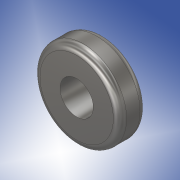
# Autodesk Inventor part: 10x26x8 Bearing
Saved by Autodesk Inventor 2017 SP1 (Build 210196100, 196)
## iProperties
Created: 2017-07-03
Part Number: 10x26x8 Bearing
Material: Steel, Carbon
Document SubType Name: Modeling
Designer: Zach
Density: 7.85 g/cm^3
Appearance: Semi-Polished
Author: Zach
Autodesk Inventor part; units mm, degrees
ref_plane "YZ Plane" through (0, 0, 0) normal (1, 0, 0) x (0, 1, 0)
ref_plane "XZ Plane" through (0, 0, 0) normal (0, 1, 0) x (-1, 0, 0)
ref_plane "XY Plane" through (0, 0, 0) normal (0, 0, 1) x (1, 0, 0)
sketch "Sketch1" plane through (0, 0, 0) normal (0, 0, 1) x (1, 0, 0)
  circle A0 centre (0, 0) radius 13
  circle A1 centre (0, 0) radius 5
  dimension "d0" = 26
  dimension "d1" = 10
  constraints: 2 centre point, 2 coincident
  measures "d0" diameter of A0
  measures "d1" diameter of A1
extrude "Extrusion1" add sketch "Sketch1" along normal blind 8
fillet "Fillet1" radius 2 2 edges at (-13, 0, 8) (-13, 0, 0)
body "Solid1"
